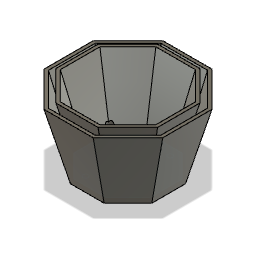
PortamacetasFinal (Autodesk Fusion 360 design; units mm, degrees)
Autodesk Fusion 360 part; units mm, degrees
sketch "Boceto1" plane through (0, 0, 0) normal (0, 1, 0) x (1, 0, 0)
  line L0 (0, 0) -> (39, 0)
  line L1 (39, 0) -> (66.5555, -27.5988)
  line L2 (66.5555, -27.5988) -> (66.5555, -66.5988)
  line L3 (66.5555, -66.5988) -> (38.9799, -94.1744)
  line L4 (38.9799, -94.1744) -> (-0.0201, -94.1744)
  line L5 (-0.0201, -94.1744) -> (-27.5719, -66.6226)
  line L6 (-27.5719, -66.6226) -> (-27.5719, -27.6226)
  line L7 (0, 0) -> (-27.5719, -27.6226)
  dimension "d1" = 39
  dimension "d11" = 45
  dimension "d14" = 45
  dimension "d15" = 39
  constraint coincident L0.start L7.start
  constraint horizontal L0
  constraint perpendicular L0 L2
  constraint horizontal L4
  constraint vertical L6
  measures "d1" distance of L0.start L0.end
  measures "d11" angle of L2 L3
  measures "d14" angle of L4 L5
  measures "d15" distance of L5.end L6.end
extrude "Extruir1" add sketch "Boceto1" along normal blind 81 draft 15 makes body 1
sketch "Boceto2" plane through (0, 81, 0) normal (0, 1, 0) x (-1, 0, 0)
  line L0 (-88.2594, 18.6188) -> (-48, -21.7039)
  line L1 (-48, -21.7039) -> (9.0017, -21.7039)
  line L2 (9.0017, -21.7039) -> (49.2757, 18.6442)
  line L3 (49.2757, 18.6442) -> (49.2757, 75.6126)
  line L4 (49.2757, 75.6126) -> (9.0101, 115.8783)
  line L5 (9.0101, 115.8783) -> (-47.97, 115.8783)
  line L6 (-47.97, 115.8783) -> (-88.2594, 75.5889)
  line L7 (-88.2594, 75.5889) -> (-88.2594, 18.6188)
  line L8 (-84.5636, 74.0587) -> (-46.4396, 112.1826)
  line L9 (-46.4396, 112.1826) -> (7.4789, 112.183)
  line L10 (7.4789, 112.183) -> (45.5805, 74.0813)
  line L11 (45.5805, 74.0813) -> (45.58, 20.1744)
  line L12 (45.58, 20.1744) -> (7.4714, -18.0082)
  line L13 (7.4714, -18.0082) -> (-46.4688, -18.0086)
  line L14 (-46.4688, -18.0086) -> (-84.5641, 20.1501)
  line L15 (-84.5641, 20.1501) -> (-84.5636, 74.0587)
  dimension "d37" = 4
  dimension "d38" = 4
  dimension "d39" = 4
  dimension "d40" = 4
  dimension "d41" = 4
  dimension "d42" = 4
  dimension "d43" = 4
  dimension "d44" = 4
  measures "d37" distance of L0.start L14.end
  measures "d38" distance of L0.end L13.end
  measures "d39" distance of L1.end L12.end
  measures "d40" distance of L2.end L11.end
  measures "d41" distance of L3.end L10.end
  measures "d42" distance of L4.end L9.end
  measures "d43" distance of L5.end L8.end
  measures "d44" distance of L6.end L8.start
extrude "Extruir2" cut sketch "Boceto2" against normal blind 77 draft -15 contours L8 L9 L10 L11 L12 L13 L14 L15 bodies 1
sketch "Boceto3" plane through (0, 0, 0) normal (0, 1, 0) x (1, 0, 0)
  circle A0 centre (51.6301, -60.3842) radius 5
  circle A1 centre (-12.5804, -33.829) radius 5
  circle A2 centre (51.6301, -60.3842) radius 5
  dimension "d49" = 10
  dimension "d50" = 10
  constraint concentric A0 A2
  measures "d49" diameter of A0
  measures "d50" diameter of A1
extrude "Extruir3" cut sketch "Boceto3" along normal blind 6 contours A0 A2 bodies 1
sketch "Boceto4" plane through (0, 0, 0) normal (0, 1, 0) x (1, 0, 0)
  circle A0 centre (51.6301, -60.3842) radius 5.0474
  circle A1 centre (51.6301, -60.3842) radius 5
  circle A2 centre (51.6301, -60.3842) radius 5
  constraint concentric A0 A1
  constraint concentric A0 A2
extrude "Extruir4" add sketch "Boceto4" along normal blind 12 contours A1 A2 bodies 1
sketch "Boceto5" plane through (0, 0, 0) normal (0, 1, 0) x (1, 0, 0)
  line L0 (-27.5719, -27.6226) -> (-15.2042, -32.7438)
  circle A0 centre (-15.2042, -32.7438) radius 5
  point P0 (66.5555, -66.5988)
  point P1 (-27.5719, -27.6226)
  dimension "d55" = 13.386
  dimension "d56" = 10
  constraint coincident P1 L0.start
  constraint coincident L0.end A0.centre
  measures "d55" distance of P1 L0.end
  measures "d56" diameter of A0
extrude "Extruir5" cut sketch "Boceto5" along normal blind 4 bodies 1
sketch "Boceto6" plane through (0, 0, 0) normal (0, 1, 0) x (1, 0, 0)
  circle A0 centre (-15.2042, -32.7438) radius 5
  circle A1 centre (-15.2042, -32.7438) radius 5
  dimension "d59" = 10
  constraint concentric A0 A1
  measures "d59" diameter of A0
extrude "Extruir6" add sketch "Boceto6" along normal blind 12 bodies 1
sketch "Boceto7" plane through (0, 0, 0) normal (0, 1, 0) x (1, 0, 0)
  circle A0 centre (5.0972, -81.8058) radius 3
  circle A1 centre (33.8751, -12.3661) radius 3
  dimension "d64" = 6
  dimension "d65" = 6
  measures "d64" diameter of A0
  measures "d65" diameter of A1
extrude "Extruir7" cut sketch "Boceto7" along normal blind 4 contours A0 bodies 1
sketch "Boceto8" plane through (0, 0, 0) normal (0, 1, 0) x (1, 0, 0)
  circle A0 centre (33.8761, -12.3665) radius 3
  point P0 (-0.0201, -94.1744)
  point P1 (39, 0)
  dimension "d68" = 13.386
  dimension "d69" = 6
  measures "d68" distance of P1 A0.centre
  measures "d69" diameter of A0
extrude "Extruir8" cut sketch "Boceto8" along normal blind 4 bodies 1
sketch "Boceto9" plane through (0, 4, 0) normal (0, 1, 0) x (-1, 0, 0)
  circle A0 centre (-33.8761, 12.3665) radius 3
  circle A1 centre (-5.0972, 81.8058) radius 3
  circle A2 centre (15.2042, 32.7438) radius 5
  circle A3 centre (-51.6301, 60.3842) radius 5
  line L0 (-37.9127, 2.6236) -> (-1.0865, 2.6238)
  line L1 (-1.0865, 2.6238) -> (24.948, 28.7089)
  line L2 (24.948, 28.7089) -> (24.9483, 65.5353)
  line L3 (24.9483, 65.5353) -> (-1.0672, 91.5508)
  line L4 (-1.0672, 91.5508) -> (-37.8935, 91.5506)
  line L5 (-37.8935, 91.5506) -> (-63.9316, 65.5125)
  line L6 (-63.9316, 65.5125) -> (-63.9319, 28.6861)
  line L7 (-63.9319, 28.6861) -> (-37.9127, 2.6236)
  circle A4 through (-30.8761, 12.3665, -4) (-35.3761, 14.9646, -4) (-35.3761, 9.7684, -4)
  circle A5 through (-30.8761, 12.3665, -4) (-35.3761, 14.9646, -4) (-35.3761, 9.7684, -4)
extrude "Extruir9" add sketch "Boceto9" along normal blind 8 contours A4 A5 in plane through (0, 0, 0) normal (0, 1, 0) bodies 1
sketch "Boceto10" plane through (0, 0, 0) normal (0, 1, 0) x (1, 0, 0)
  circle A0 centre (5.0972, -81.8058) radius 3
  circle A1 centre (5.0972, -81.8058) radius 3
  dimension "d74" = 6
  constraint concentric A0 A1
  measures "d74" diameter of A0
extrude "Extruir10" add sketch "Boceto10" along normal blind 8 bodies 1
sketch "Boceto11" plane through (0, 4, 0) normal (0, 1, 0) x (-1, 0, 0)
  circle A0 centre (-33.8761, 12.3665) radius 3
  circle A1 centre (-5.0972, 81.8058) radius 3
  circle A2 centre (15.2042, 32.7438) radius 5
  circle A3 centre (-51.6301, 60.3842) radius 5
  line L0 (-37.9127, 2.6236) -> (-1.0865, 2.6238)
  line L1 (-1.0865, 2.6238) -> (24.948, 28.7089)
  line L2 (24.948, 28.7089) -> (24.9483, 65.5353)
  line L3 (24.9483, 65.5353) -> (-1.0672, 91.5508)
  line L4 (-1.0672, 91.5508) -> (-37.8935, 91.5506)
  line L5 (-37.8935, 91.5506) -> (-63.9316, 65.5125)
  line L6 (-63.9316, 65.5125) -> (-63.9319, 28.6861)
  line L7 (-63.9319, 28.6861) -> (-37.9127, 2.6236)
  line L8 (-195, 0) -> (-226.935, 0)
  line L9 (-226.935, 0) -> (-249.5165, 22.5815)
  line L10 (-249.5165, 22.5815) -> (-249.5165, 54.5165)
  line L11 (-249.5165, 54.5165) -> (-226.935, 77.0979)
  line L12 (-226.935, 77.0979) -> (-195, 77.0979)
  line L13 (-195, 77.0979) -> (-172.4185, 54.5165)
  line L14 (-172.4185, 54.5165) -> (-172.4185, 22.5815)
  line L15 (-172.4185, 22.5815) -> (-195, 0)
  constraint horizontal L8
  constraint vertical L10
  constraint horizontal L12
  constraint vertical L14
extrude "Extruir11" add sketch "Boceto11" along normal blind 76.172 draft 15 separate body contours L8 L9 L10 L11 L12 L13 L14 L15 makes body 2
sketch "Boceto12" plane through (0, 0, 0) normal (0, 1, 0) x (1, 0, 0)
  line L0 (188.0765, -93.8126, 80.172) -> (233.8585, -93.8126, 80.172)
  line L1 (233.8585, -93.8126, 80.172) -> (266.2312, -61.4399, 80.172)
  line L2 (266.2312, -61.4399, 80.172) -> (266.2312, -15.658, 80.172)
  line L3 (266.2312, -15.658, 80.172) -> (233.8585, 16.7147, 80.172)
  line L4 (233.8585, 16.7147, 80.172) -> (188.0765, 16.7147, 80.172)
  line L5 (188.0765, 16.7147, 80.172) -> (155.7038, -15.658, 80.172)
  line L6 (155.7038, -15.658, 80.172) -> (155.7038, -61.4399, 80.172)
  line L7 (155.7038, -61.4399, 80.172) -> (188.0765, -93.8126, 80.172)
  point P0 (235.3892, -97.5081)
  point P1 (186.5458, 20.4102)
  point P2 (269.9267, -62.9706)
  point P3 (152.0083, -14.1273)
  point P4 (269.9267, -14.1273)
  point P5 (152.0083, -62.9706)
  point P6 (186.5458, -97.5081)
  point P7 (235.3892, 20.4102)
  point P8 (172.4185, -22.5815)
  dimension "d98" = 4
  dimension "d99" = 4
  dimension "d100" = 4
  dimension "d101" = 4
  dimension "d103" = 4
  dimension "d104" = 4
  dimension "d105" = 4
  dimension "d106" = 4
  dimension "d107" = 77.9843
extrude "Extruir12" cut sketch "Boceto12" against normal blind 75.311 draft -15 contours L0 L1 L2 L3 L4 L5 L6 L7 in plane through (0, 80.172, 0) normal (0, 1, 0) bodies 2
sketch "Boceto13" plane through (0, 4, 0) normal (0, 1, 0) x (-1, 0, 0)
  circle A0 centre (-33.8761, 12.3665) radius 3
  circle A1 centre (-5.0972, 81.8058) radius 3
  circle A2 centre (15.2042, 32.7438) radius 5
  circle A3 centre (-51.6301, 60.3842) radius 5
  line L0 (-37.9127, 2.6236) -> (-1.0865, 2.6238)
  line L1 (-1.0865, 2.6238) -> (24.948, 28.7089)
  line L2 (24.948, 28.7089) -> (24.9483, 65.5353)
  line L3 (24.9483, 65.5353) -> (-1.0672, 91.5508)
  line L4 (-1.0672, 91.5508) -> (-37.8935, 91.5506)
  line L5 (-37.8935, 91.5506) -> (-63.9316, 65.5125)
  line L6 (-63.9316, 65.5125) -> (-63.9319, 28.6861)
  line L7 (-63.9319, 28.6861) -> (-37.9127, 2.6236)
  line L8 (-249.5165, 54.5165) -> (-244.594, 52.4775)
  circle A4 centre (-177.341, 24.6204) radius 5
  point P0 (-249.5165, 54.5165)
  point P1 (-172.4185, 22.5815)
  dimension "d111" = 5.328
  dimension "d112" = 5.328
  dimension "d113" = 10
  constraint coincident P0 L8.start
  measures "d111" distance of P0 L8.end
  measures "d112" distance of P1 A4.centre
  measures "d113" diameter of A4
extrude "Extruir13" cut sketch "Boceto13" along normal blind 17 contours A4 bodies 2
sketch "Boceto14" plane through (0, 4, 0) normal (0, -1, 0) x (1, 0, 0)
  arc A0 (174.4806, 20.5194) -> (172.4185, 25.4977) centre (177.341, 24.6204) ccw
  line L0 (174.4806, 20.5194) -> (195, 0)
  line L1 (195, 0) -> (226.935, 0)
  line L2 (226.935, 0) -> (249.5165, 22.5815)
  line L3 (249.5165, 22.5815) -> (249.5165, 54.5165)
  line L4 (249.5165, 54.5165) -> (226.935, 77.0979)
  line L5 (226.935, 77.0979) -> (195, 77.0979)
  line L6 (195, 77.0979) -> (172.4185, 54.5165)
  line L7 (172.4185, 54.5165) -> (172.4185, 25.4977)
  circle A1 centre (244.594, 52.4775) radius 5
  dimension "d116" = 5.328
  dimension "d117" = 10
  measures "d116" distance of L3.end A1.centre
  measures "d117" diameter of A1
extrude "Extruir14" cut sketch "Boceto14" against normal blind 30 contours L3 L4 A1 picked at (246.477, 50.9898) bodies 2
sketch "Boceto15" plane through (0, 4, 0) normal (0, 1, 0) x (-1, 0, 0)
  circle A0 centre (-33.8761, 12.3665) radius 3
  circle A1 centre (-5.0972, 81.8058) radius 3
  line L0 (-37.9127, 2.6236) -> (-1.0865, 2.6238)
  line L1 (-1.0865, 2.6238) -> (24.948, 28.7089)
  line L2 (24.948, 28.7089) -> (24.9483, 65.5353)
  line L3 (24.9483, 65.5353) -> (-1.0672, 91.5508)
  line L4 (-1.0672, 91.5508) -> (-37.8935, 91.5506)
  line L5 (-37.8935, 91.5506) -> (-63.9316, 65.5125)
  line L6 (-63.9316, 65.5125) -> (-63.9319, 28.6861)
  line L7 (-63.9319, 28.6861) -> (-37.9127, 2.6236)
sketch "Boceto16" plane through (0, 0, 0) normal (0, 0, 1) x (1, 0, 0)
sketch "Boceto17" plane through (0, 0, 0) normal (0, 0, 1) x (1, 0, 0)
extrude "Extruir15" cut 1 faces at (-14.1651, 12, 30.4582) along direction (0, -1, 0) blind 8 on bodies 1 bodies 1
extrude "Extruir16" cut 1 faces at (53.1722, 12, 62.0462) along direction (0, -1, 0) blind 8 on bodies 1 bodies 1
sketch "Boceto18" plane through (0, 0, 0) normal (0, -1, 0) x (1, 0, 0)
  line L0 (0, 0) -> (39, 0)
  line L1 (39, 0) -> (66.5555, 27.5988)
  line L2 (66.5555, 27.5988) -> (66.5555, 66.5988)
  line L3 (66.5555, 66.5988) -> (38.9799, 94.1744)
  line L4 (38.9799, 94.1744) -> (-0.0201, 94.1744)
  line L5 (-0.0201, 94.1744) -> (-27.5719, 66.6226)
  line L6 (-27.5719, 66.6226) -> (-27.5719, 27.6226)
  line L7 (-27.5719, 27.6226) -> (0, 0)
  circle A0 centre (53.1198, 61.0354) radius 5
  circle A1 centre (-14.1362, 33.186) radius 5
  dimension "d126" = 10
  dimension "d127" = 10
  measures "d126" diameter of A0
  measures "d127" diameter of A1
extrude "Extruir17" cut sketch "Boceto18" against normal blind 15 contours A0 bodies 1
sketch "Boceto19" plane through (0, 0, 0) normal (0, 1, 0) x (1, 0, 0)
  circle A0 centre (-14.1158, -33.1883) radius 5
  dimension "d131" = 10
  measures "d131" diameter of A0
extrude "Extruir18" cut sketch "Boceto19" along normal blind 9 bodies 1
sketch "Boceto20" plane through (0, 0, 0) normal (0, -1, 0) x (1, 0, 0)
  circle A0 centre (-14.1158, 33.1883) radius 5
  circle A1 centre (53.1198, 61.0354) radius 5
  line L0 (0, 0) -> (39, 0)
  line L1 (39, 0) -> (66.5555, 27.5988)
  line L2 (66.5555, 27.5988) -> (66.5555, 66.5988)
  line L3 (66.5555, 66.5988) -> (38.9799, 94.1744)
  line L4 (38.9799, 94.1744) -> (-0.0201, 94.1744)
  line L5 (-0.0201, 94.1744) -> (-27.5719, 66.6226)
  line L6 (-27.5719, 66.6226) -> (-27.5719, 27.6226)
  line L7 (-27.5719, 27.6226) -> (0, 0)
  circle A2 centre (-14.1158, 33.1883) radius 5
  constraint concentric A0 A2
extrude "Extruir19" add sketch "Boceto20" against normal blind 12 contours A0 A2 bodies 1
sketch "Boceto21" plane through (0, 0, 0) normal (0, -1, 0) x (1, 0, 0)
  circle A0 centre (53.1198, 61.0354) radius 5
  line L0 (0, 0) -> (39, 0)
  line L1 (39, 0) -> (66.5555, 27.5988)
  line L2 (66.5555, 27.5988) -> (66.5555, 66.5988)
  line L3 (66.5555, 66.5988) -> (38.9799, 94.1744)
  line L4 (38.9799, 94.1744) -> (-0.0201, 94.1744)
  line L5 (-0.0201, 94.1744) -> (-27.5719, 66.6226)
  line L6 (-27.5719, 66.6226) -> (-27.5719, 27.6226)
  line L7 (-27.5719, 27.6226) -> (0, 0)
  circle A1 centre (53.1198, 61.0354) radius 5
  constraint concentric A0 A1
extrude "Extruir20" add sketch "Boceto21" against normal blind 12 contours A0 A1 bodies 1
move_body "Desplazar1" bodies 2 to x (1, 0, 0) y (0, 1, 0) z (0, 0, 1) at (-191.754, 4.1024, 8.4099)
